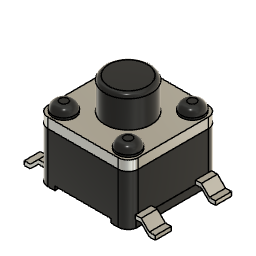
Tac Switch_4.5mm_H4.3mm (Autodesk Fusion 360 design; units mm, degrees)
Autodesk Fusion 360 part; units mm, degrees
sketch "Sketch1" plane through (0, 0, 0) normal (0, 0, 1) x (1, 0, 0)
  line L0 (2.25, -2.25) -> (-2.25, -2.25)
  line L1 (-2.25, -2.25) -> (-2.25, 2.25)
  line L2 (-2.25, 2.25) -> (2.25, 2.25)
  line L3 (2.25, 2.25) -> (2.25, -2.25)
  line L4 (2.25, -2.25) -> (-2.25, 2.25) construction
  line L5 (-2.25, -2.25) -> (2.25, 2.25) construction
  dimension "d1" = 4.5
  dimension "d2" = 4.5
  constraint horizontal L0
  constraint perpendicular L0 L1
  constraint parallel L0 L2
  constraint parallel L1 L3
  constraint coincident L4 origin
  constraint coincident L5 origin
  measures "d1" distance of L1.end L2.end
  measures "d2" distance of L0.end L1.end
extrude "Extrude1" add sketch "Sketch1" along normal blind 2.5 makes body 1
extrude "Extrude2" add 1 faces at (0.75, -0.75, 2.5) along direction (0, 0, 1) blind 0.5 separate body on bodies 1 makes body 2
sketch "Sketch2" plane through (0, 0, 3) normal (0, 0, 1) x (-1, 0, 0)
  line L0 (-2.25, -2.25) -> (2.25, -2.25)
  line L1 (2.25, -2.25) -> (2.25, 2.25)
  line L2 (2.25, 2.25) -> (-2.25, 2.25)
  line L3 (-2.25, 2.25) -> (-2.25, -2.25)
  circle A0 centre (0, 0) radius 1.15
  circle A1 centre (1.6, -1.6) radius 0.55
  circle A2 centre (-1.6, -1.6) radius 0.55
  circle A3 centre (1.6, 1.6) radius 0.55
  circle A4 centre (-1.6, 1.6) radius 0.55
  dimension "d7" = 2.3
  dimension "d8" = 1.1
  dimension "d9" = 0.65
  dimension "d10" = 0.65
  dimension "d13" = -3.2
  dimension "d14" = 3.2
  constraint coincident A0.centre origin
  measures "d7" diameter of A0
  measures "d8" diameter of A1
  measures "d9" distance of L0 A1.centre
  measures "d10" distance of L1 A1.centre
extrude "Extrude3" add sketch "Sketch2" along normal blind 1.55 separate body contours A0 makes body 3
extrude "Extrude4" add sketch "Sketch2" along normal blind 0.45 separate body contours A1 | A2 | A3 | A4 makes body 4 at (-2.1473, 1.6548, 3.15) makes body 5 at (1.0527, 1.6548, 3.15) makes body 6 at (-2.1473, -1.5452, 3.15) makes body 7 at (1.0527, -1.5452, 3.15)
fillet "Fillet1" radius 0.5 8 edges at (2.25, -2.25, 1.25) (-2.25, -2.25, 1.25) (-2.25, 2.25, 1.25) (2.25, 2.25, 1.25) (2.25, -2.25, 2.75) (-2.25, -2.25, 2.75) (-2.25, 2.25, 2.75) (2.25, 2.25, 2.75) on bodies 1 2
fillet "Fillet2" radius 0.35 4 edges at (-1.0872, 1.7989, 3.45) (2.1128, 1.7989, 3.45) (-1.0872, -1.4011, 3.45) (2.1128, -1.4011, 3.45) on bodies 4 5 6 7
fillet "Fillet3" radius 0.2 1 edges at (1.0722, 0.4159, 4.55) on bodies 3
sketch "Sketch3" plane through (0, -2.25, 0) normal (0, -1, 0) x (1, 0, 0)
  line L0 (-1.75, 2.5) -> (-1.75, 0)
  line L1 (-1.75, 0) -> (1.75, 0)
  line L2 (1.75, 0) -> (1.75, 2.5)
  line L3 (1.75, 2.5) -> (-1.75, 2.5)
  line L4 (1.4, 0.2) -> (-1.4, 0.2)
  line L5 (-1.4, 0.2) -> (-1.4, 0)
  line L6 (1.4, 0) -> (1.4, 0.2)
  constraint horizontal L4
  constraint perpendicular L4 L5
  constraint parallel L5 L6
  constraint coincident L1 L5.end
  constraint coincident L1 L6.start
extrude "Extrude5" cut sketch "Sketch3" against normal blind 4.5 contours L1 L4 L5 L6 bodies 1
sketch "Sketch4" plane through (0, 0, 0) normal (0, 0, 1) x (1, 0, 0)
  line L0 (-2.2533, 2.6048) -> (-2.2533, -2.6449) construction
  line L1 (3.1297, -2.259) -> (-2.9, -2.259) construction
  line L2 (-2.2533, -0.0201) -> (-2.2533, 1.4799) construction
  line L3 (-2.2533, -0.0201) -> (-2.2533, -1.5201) construction
  line L4 (2.2406, 0.0108) -> (2.2406, 1.5108) construction
  line L5 (2.2406, 0.0108) -> (2.2406, -1.4892) construction
  line L6 (-3.2533, 1.8799) -> (-2.2533, 1.8799)
  line L7 (-2.2533, 1.8799) -> (-2.2533, 1.0799)
  line L8 (-2.2533, 1.0799) -> (-3.2533, 1.0799)
  line L9 (-3.2533, 1.0799) -> (-3.2533, 1.8799)
  line L10 (-2.2533, 1.0799) -> (-3.2533, 1.8799) construction
  line L11 (-3.2533, 1.0799) -> (-2.2533, 1.8799) construction
  line L12 (-2.7533, 1.4799) -> (-3.2533, 1.4799) construction
  line L13 (-3.2533, 1.4799) -> (-2.7533, 1.4799) construction
  line L14 (-2.7533, 1.4799) -> (-2.2533, 1.4799) construction
  line L15 (3.2406, -1.0892) -> (3.2406, -1.8892)
  line L16 (2.2406, -1.8892) -> (3.2406, -1.0892) construction
  line L17 (2.2406, -1.4892) -> (2.7406, -1.4892) construction
  line L18 (2.7406, -1.4892) -> (2.2406, -1.4892) construction
  line L19 (2.7406, -1.4892) -> (3.2406, -1.4892) construction
  line L20 (3.2406, -1.8892) -> (2.2406, -1.8892)
  line L21 (3.2406, -1.8892) -> (2.2406, -1.0892) construction
  line L22 (2.2406, -1.8892) -> (2.2406, -1.0892)
  line L23 (2.2406, -1.0892) -> (3.2406, -1.0892)
  line L24 (2.2406, 1.5108) -> (2.7406, 1.5108) construction
  line L25 (3.2406, 1.9108) -> (3.2406, 1.1108)
  line L26 (2.7406, 1.5108) -> (3.2406, 1.5108) construction
  line L27 (2.2406, 1.1108) -> (3.2406, 1.9108) construction
  line L28 (3.2406, 1.1108) -> (2.2406, 1.9108) construction
  line L29 (3.2406, 1.1108) -> (2.2406, 1.1108)
  line L30 (2.2406, 1.1108) -> (2.2406, 1.9108)
  line L31 (2.2406, 1.9108) -> (3.2406, 1.9108)
  line L32 (2.7406, 1.5108) -> (2.2406, 1.5108) construction
  line L33 (-2.2533, -1.1201) -> (-2.2533, -1.9201)
  line L34 (-3.2533, -1.1201) -> (-2.2533, -1.1201)
  line L35 (-2.7533, -1.5201) -> (-2.2533, -1.5201) construction
  line L36 (-3.2533, -1.9201) -> (-2.2533, -1.1201) construction
  line L37 (-2.2533, -1.9201) -> (-3.2533, -1.1201) construction
  line L38 (-2.2533, -1.9201) -> (-3.2533, -1.9201)
  line L39 (-2.7533, -1.5201) -> (-3.2533, -1.5201) construction
  line L40 (-3.2533, -1.5201) -> (-2.7533, -1.5201) construction
  line L41 (-3.2533, -1.9201) -> (-3.2533, -1.1201)
  dimension "d27" = 1.5
  dimension "d28" = 1.5
  dimension "d29" = 1.5
  dimension "d30" = 1.5
  dimension "d31" = 1
  dimension "d32" = 0.8
  dimension "d33" = 1
  dimension "d34" = 0.8
  dimension "d35" = 1
  dimension "d36" = 0.8
  dimension "d37" = 1
  dimension "d38" = 0.8
  constraint vertical L0
  constraint perpendicular L0 L1
  constraint midpoint L0 L2.start
  constraint parallel L0 L2
  constraint parallel L0 L3
  constraint vertical L4
  constraint parallel L4 L5
  constraint horizontal L6
  constraint vertical L7
  constraint horizontal L8
  constraint vertical L9
  constraint midpoint L11 L12.start
  constraint midpoint L9 L12.end
  constraint midpoint L7 L2.end
  constraint horizontal L23
  constraint vertical L15
  constraint horizontal L20
  constraint vertical L22
  constraint midpoint L17.end L16
  constraint midpoint L5.end L22
  constraint midpoint L19.end L15
  constraint horizontal L31
  constraint vertical L25
  constraint horizontal L29
  constraint vertical L30
  constraint midpoint L24.end L27
  constraint midpoint L4.end L30
  constraint midpoint L26.end L25
  constraint horizontal L34
  constraint vertical L33
  constraint horizontal L38
  constraint vertical L41
  constraint midpoint L35.start L36
  constraint midpoint L39.end L41
  constraint midpoint L3.end L33
  measures "d27" distance of L2.start L2.end
  measures "d28" distance of L2.start L3.end
  measures "d29" distance of L4.start L4.end
  measures "d30" distance of L4.start L5.end
  measures "d31" distance of L6.start L6.end
  measures "d32" distance of L6.start L8.end
  measures "d33" distance of L21.end L15.start
  measures "d34" distance of L21.end L16.start
  measures "d35" distance of L28.end L25.start
  measures "d36" distance of L28.end L27.start
  measures "d37" distance of L34.start L33.start
  measures "d38" distance of L34.start L36.start
extrude "Extrude6" add sketch "Sketch4" along normal blind 0.6 separate body makes body 8 at (-2.9199, -1.6534, 0) makes body 9 at (2.9073, -1.6226, 0) makes body 10 at (-2.9199, 1.3466, 0) makes body 11 at (2.574, 1.6441, 0)
sketch "Sketch5" plane through (0, -1.8892, 0) normal (0, -1, 0) x (1, 0, 0)
  line L0 (2.2406, 0) -> (3.2406, 0)
  line L1 (3.2406, 0) -> (3.2406, 0.6)
  line L2 (3.2406, 0.6) -> (2.2406, 0.6)
  line L3 (2.2406, 0.6) -> (2.2406, 0)
  line L4 (3.2406, 0.6) -> (2.9406, 0.6)
  line L5 (2.9406, 0.6) -> (2.9406, 0.2)
  line L6 (2.9406, 0.2) -> (3.2406, 0.2)
  line L7 (3.2406, 0.2) -> (3.2406, 0.6)
  line L8 (2.2406, 0) -> (2.5406, 0)
  line L9 (2.5406, 0) -> (2.5406, 0.4)
  line L10 (2.5406, 0.4) -> (2.2406, 0.4)
  line L11 (2.2406, 0.4) -> (2.2406, 0)
  dimension "d41" = 0.3
  dimension "d42" = 0.4
  dimension "d43" = 0.3
  dimension "d44" = 0.4
  constraint horizontal L4
  constraint vertical L5
  constraint horizontal L6
  constraint vertical L7
  constraint coincident L1.end L2.start
  constraint horizontal L8
  constraint vertical L9
  constraint horizontal L10
  constraint vertical L11
  constraint coincident L0.start L3.end
  measures "d41" distance of L1.end L4.end
  measures "d42" distance of L1.end L6.end
  measures "d43" distance of L0.start L8.end
  measures "d44" distance of L0.start L10.end
extrude "Extrude7" cut sketch "Sketch5" against normal blind 4.5 contours L0 L3 L8 L9 L10 L11 | L1 L2 L4 L5 L6 L7 bodies 1 9 11
sketch "Sketch6" plane through (0, -1.9201, 0) normal (0, -1, 0) x (1, 0, 0)
  line L0 (-3.2533, 0) -> (-2.2533, 0)
  line L1 (-2.2533, 0) -> (-2.2533, 0.6)
  line L2 (-2.2533, 0.6) -> (-3.2533, 0.6)
  line L3 (-3.2533, 0.6) -> (-3.2533, 0)
  line L4 (-3.2533, 0.6) -> (-2.9533, 0.6)
  line L5 (-2.9533, 0.6) -> (-2.9533, 0.2)
  line L6 (-2.9533, 0.2) -> (-3.2533, 0.2)
  line L7 (-3.2533, 0.2) -> (-3.2533, 0.6)
  line L8 (-2.2533, 0) -> (-2.5533, 0)
  line L9 (-2.5533, 0) -> (-2.5533, 0.4)
  line L10 (-2.5533, 0.4) -> (-2.2533, 0.4)
  line L11 (-2.2533, 0.4) -> (-2.2533, 0)
  dimension "d47" = 0.3
  dimension "d48" = 0.4
  dimension "d49" = 0.3
  dimension "d50" = 0.4
  constraint horizontal L4
  constraint vertical L5
  constraint horizontal L6
  constraint vertical L7
  constraint coincident L2.end L3.start
  constraint horizontal L8
  constraint vertical L9
  constraint horizontal L10
  constraint vertical L11
  constraint coincident L0.end L1.start
  measures "d47" distance of L2.end L4.end
  measures "d48" distance of L2.end L6.end
  measures "d49" distance of L0.end L8.end
  measures "d50" distance of L0.end L10.end
extrude "Extrude8" cut sketch "Sketch6" against normal blind 4.5 contours L0 L1 L8 L9 L10 L11 | L2 L3 L4 L5 L6 L7 bodies 8 10
chamfer "Chamfer1" distance 0.4 angle 45 8 edges at (-2.9533, 1.4799, 0.6) (-2.5533, 1.4799, 0) (-2.9533, -1.5201, 0.6) (-2.5533, -1.5201, 0) (2.9406, 1.5108, 0.6) (2.5406, 1.5108, 0) (2.9406, -1.4892, 0.6) (2.5406, -1.4892, 0) on bodies 8 9 10 11
